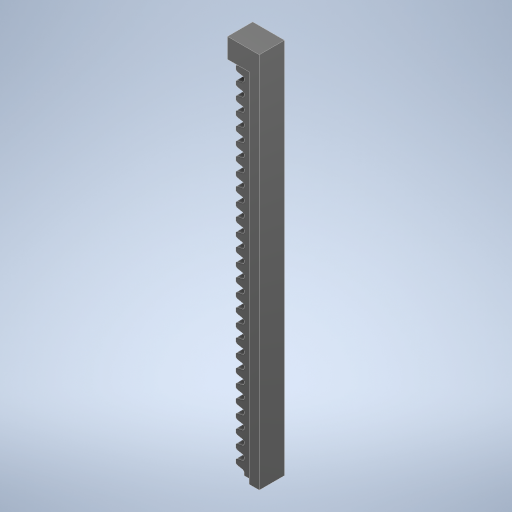
# Autodesk Inventor part: Hreben_Stylus
Saved by Autodesk Inventor 2024.2 (Build 282272000, 272)
## iProperties
Created: 2025-06-02
Part Number: Hreben_Stylus
Material: Termoplastická pryskyřice
Document SubType Name: Modeling
Designer: Elite
Density: 1.28 g/cm^3
Appearance: Hladká – černá
Mass: 4.51235 g
Surface Area: 29.4448 cm^2
Volume: 3.52528 cm^3
Author: Elite
Autodesk Inventor part; units mm, degrees
ref_plane "YZ Plane" through (0, 0, 0) normal (1, 0, 0) x (0, 1, 0)
ref_plane "XZ Plane" through (0, 0, 0) normal (0, 1, 0) x (-1, 0, 0)
ref_plane "XY Plane" through (0, 0, 0) normal (0, 0, 1) x (1, 0, 0)
sketch "Náčrt1" plane through (0, 0, 0) normal (0, 0, 1) x (1, 0, 0)
  line L0 (-2.539999, 6.35) -> (0, 6.35)
  line L1 (-2.539999, 6.35) -> (-3.809999, 5.08)
  line L2 (-3.809999, 5.08) -> (-5.079999, 5.08)
  line L3 (-5.079999, 5.08) -> (-5.079999, 1.27)
  line L4 (-5.079999, 1.27) -> (-3.809999, 1.27)
  line L5 (-3.809999, 1.27) -> (-2.539999, 0)
  line L6 (-2.539999, 0) -> (0, 0)
  line L7 (0, 0) -> (0, 6.35)
  constraints: 16 end point
extrude "Vysunutí1" add sketch "Náčrt1" against normal blind 90
sketch "Náčrt2" plane through (-3.809999, 5.08, 0) normal (0, 1, 0) x (1, 0, 0)
  line L0 (0, 0) -> (-1.27, 0)
  line L1 (0, 0) -> (0, 90)
  line L2 (-1.27, 90) -> (0, 90)
  line L3 (-1.27, 0) -> (-1.27, 90)
  arc A0 (-1.678461, 2.998415) -> (-1.27, 3.497336) centre (-1.778009, 3.496575) ccw
  arc A1 (-2.97646, 2.739034) -> (-3.389, 2.240304) centre (-2.881172, 2.240226) ccw
  arc A2 (-3.389, 1.845748) -> (-2.971901, 1.32351) centre (-2.881505, 1.82339) ccw
  line L4 (-2.990322, 1.327194) -> (-2.971901, 1.32351)
  arc A3 (-1.27, 0.566986) -> (-1.677758, 1.064456) centre (-1.777338, 0.566986) ccw
  line L5 (-1.27, 3.868884) -> (-1.27, 3.495814)
  line L6 (-1.27, 0) -> (-1.27, 90)
  line L7 (-2.971901, 1.32351) -> (-1.677758, 1.064456)
  line L8 (-3.389, 1.845748) -> (-3.389, 2.24059)
  line L9 (-2.97646, 2.739034) -> (-1.678461, 2.998415)
  line L10 (-1.27, 0.566986) -> (-1.27, 3.868884)
  arc A4 (-1.678461, 6.300312) -> (-1.27, 6.799234) centre (-1.778009, 6.798472) ccw
  arc A5 (-2.97646, 6.040931) -> (-3.389, 5.542202) centre (-2.881172, 5.542123) ccw
  arc A6 (-3.389, 5.147645) -> (-2.971901, 4.625407) centre (-2.881505, 5.125287) ccw
  line L11 (-2.990322, 4.629092) -> (-2.971901, 4.625407)
  arc A7 (-1.27, 3.868884) -> (-1.677758, 4.366353) centre (-1.777338, 3.868884) ccw
  line L12 (-1.27, 7.170781) -> (-1.27, 6.797711)
  line L13 (-2.971901, 4.625407) -> (-1.677758, 4.366353)
  line L14 (-3.389, 5.147645) -> (-3.389, 5.542488)
  line L15 (-2.97646, 6.040931) -> (-1.678461, 6.300312)
  line L16 (-1.27, 3.868884) -> (-1.27, 7.170781)
  arc A8 (-1.678461, 9.602209) -> (-1.27, 10.101131) centre (-1.778009, 10.10037) ccw
  arc A9 (-2.97646, 9.342828) -> (-3.389, 8.844099) centre (-2.881172, 8.844021) ccw
  arc A10 (-3.389, 8.449542) -> (-2.971901, 7.927305) centre (-2.881505, 8.427184) ccw
  line L17 (-2.990322, 7.930989) -> (-2.971901, 7.927305)
  arc A11 (-1.27, 7.170781) -> (-1.677758, 7.668251) centre (-1.777338, 7.170781) ccw
  line L18 (-1.27, 10.472678) -> (-1.27, 10.099608)
  line L19 (-2.971901, 7.927305) -> (-1.677758, 7.668251)
  line L20 (-3.389, 8.449542) -> (-3.389, 8.844385)
  line L21 (-2.97646, 9.342828) -> (-1.678461, 9.602209)
  line L22 (-1.27, 7.170781) -> (-1.27, 10.472678)
  arc A12 (-1.678461, 12.904106) -> (-1.27, 13.403028) centre (-1.778009, 13.402267) ccw
  arc A13 (-2.97646, 12.644726) -> (-3.389, 12.145996) centre (-2.881172, 12.145918) ccw
  arc A14 (-3.389, 11.751439) -> (-2.971901, 11.229202) centre (-2.881505, 11.729081) ccw
  line L23 (-2.990322, 11.232886) -> (-2.971901, 11.229202)
  arc A15 (-1.27, 10.472678) -> (-1.677758, 10.970148) centre (-1.777338, 10.472678) ccw
  line L24 (-1.27, 13.774575) -> (-1.27, 13.401505)
  line L25 (-2.971901, 11.229202) -> (-1.677758, 10.970148)
  line L26 (-3.389, 11.751439) -> (-3.389, 12.146282)
  line L27 (-2.97646, 12.644726) -> (-1.678461, 12.904106)
  line L28 (-1.27, 10.472678) -> (-1.27, 13.774575)
  arc A16 (-1.678461, 16.206003) -> (-1.27, 16.704925) centre (-1.778009, 16.704164) ccw
  arc A17 (-2.97646, 15.946623) -> (-3.389, 15.447893) centre (-2.881172, 15.447815) ccw
  arc A18 (-3.389, 15.053337) -> (-2.971901, 14.531099) centre (-2.881505, 15.030979) ccw
  line L29 (-2.990322, 14.534783) -> (-2.971901, 14.531099)
  arc A19 (-1.27, 13.774575) -> (-1.677758, 14.272045) centre (-1.777338, 13.774575) ccw
  line L30 (-1.27, 17.076472) -> (-1.27, 16.703403)
  line L31 (-2.971901, 14.531099) -> (-1.677758, 14.272045)
  line L32 (-3.389, 15.053337) -> (-3.389, 15.448179)
  line L33 (-2.97646, 15.946623) -> (-1.678461, 16.206003)
  line L34 (-1.27, 13.774575) -> (-1.27, 17.076472)
  arc A20 (-1.678461, 19.507901) -> (-1.27, 20.006822) centre (-1.778009, 20.006061) ccw
  arc A21 (-2.97646, 19.24852) -> (-3.389, 18.74979) centre (-2.881172, 18.749712) ccw
  arc A22 (-3.389, 18.355234) -> (-2.971901, 17.832996) centre (-2.881505, 18.332876) ccw
  line L35 (-2.990322, 17.83668) -> (-2.971901, 17.832996)
  arc A23 (-1.27, 17.076472) -> (-1.677758, 17.573942) centre (-1.777338, 17.076472) ccw
  line L36 (-1.27, 20.37837) -> (-1.27, 20.0053)
  line L37 (-2.971901, 17.832996) -> (-1.677758, 17.573942)
  line L38 (-3.389, 18.355234) -> (-3.389, 18.750076)
  line L39 (-2.97646, 19.24852) -> (-1.678461, 19.507901)
  line L40 (-1.27, 17.076472) -> (-1.27, 20.37837)
  arc A24 (-1.678461, 22.809798) -> (-1.27, 23.30872) centre (-1.778009, 23.307958) ccw
  arc A25 (-2.97646, 22.550417) -> (-3.389, 22.051688) centre (-2.881172, 22.051609) ccw
  arc A26 (-3.389, 21.657131) -> (-2.971901, 21.134893) centre (-2.881505, 21.634773) ccw
  line L41 (-2.990322, 21.138578) -> (-2.971901, 21.134893)
  arc A27 (-1.27, 20.37837) -> (-1.677758, 20.875839) centre (-1.777338, 20.37837) ccw
  line L42 (-1.27, 23.680267) -> (-1.27, 23.307197)
  line L43 (-2.971901, 21.134893) -> (-1.677758, 20.875839)
  line L44 (-3.389, 21.657131) -> (-3.389, 22.051974)
  line L45 (-2.97646, 22.550417) -> (-1.678461, 22.809798)
  line L46 (-1.27, 20.37837) -> (-1.27, 23.680267)
  arc A28 (-1.678461, 26.111695) -> (-1.27, 26.610617) centre (-1.778009, 26.609856) ccw
  arc A29 (-2.97646, 25.852314) -> (-3.389, 25.353585) centre (-2.881172, 25.353507) ccw
  arc A30 (-3.389, 24.959028) -> (-2.971901, 24.436791) centre (-2.881505, 24.93667) ccw
  line L47 (-2.990322, 24.440475) -> (-2.971901, 24.436791)
  arc A31 (-1.27, 23.680267) -> (-1.677758, 24.177737) centre (-1.777338, 23.680267) ccw
  line L48 (-1.27, 26.982164) -> (-1.27, 26.609094)
  line L49 (-2.971901, 24.436791) -> (-1.677758, 24.177737)
  line L50 (-3.389, 24.959028) -> (-3.389, 25.353871)
  line L51 (-2.97646, 25.852314) -> (-1.678461, 26.111695)
  line L52 (-1.27, 23.680267) -> (-1.27, 26.982164)
  line L53 (-2.971901, 27.738688) -> (-1.677758, 27.479634)
  line L54 (-2.97646, 29.154212) -> (-1.678461, 29.413592)
  line L55 (-2.990322, 27.742372) -> (-2.971901, 27.738688)
  arc A32 (-2.97646, 29.154212) -> (-3.389, 28.655482) centre (-2.881172, 28.655404) ccw
  line L56 (-3.389, 28.260925) -> (-3.389, 28.655768)
  arc A33 (-3.389, 28.260925) -> (-2.971901, 27.738688) centre (-2.881505, 28.238567) ccw
  arc A34 (-1.27, 26.982164) -> (-1.677758, 27.479634) centre (-1.777338, 26.982164) ccw
  arc A35 (-1.678461, 29.413592) -> (-1.27, 29.912514) centre (-1.778009, 29.911753) ccw
  line L57 (-1.27, 30.284061) -> (-1.27, 29.910991)
  line L58 (-1.27, 26.982164) -> (-1.27, 30.284061)
  line L59 (-2.971901, 31.040585) -> (-1.677758, 30.781531)
  line L60 (-2.97646, 32.456109) -> (-1.678461, 32.715489)
  line L61 (-2.990322, 31.044269) -> (-2.971901, 31.040585)
  arc A36 (-2.97646, 32.456109) -> (-3.389, 31.957379) centre (-2.881172, 31.957301) ccw
  line L62 (-3.389, 31.562823) -> (-3.389, 31.957665)
  arc A37 (-3.389, 31.562823) -> (-2.971901, 31.040585) centre (-2.881505, 31.540465) ccw
  arc A38 (-1.27, 30.284061) -> (-1.677758, 30.781531) centre (-1.777338, 30.284061) ccw
  arc A39 (-1.678461, 32.715489) -> (-1.27, 33.214411) centre (-1.778009, 33.21365) ccw
  line L63 (-1.27, 33.585958) -> (-1.27, 33.212889)
  line L64 (-1.27, 30.284061) -> (-1.27, 33.585958)
  line L65 (-2.971901, 34.342482) -> (-1.677758, 34.083428)
  line L66 (-2.97646, 35.758006) -> (-1.678461, 36.017387)
  line L67 (-2.990322, 34.346166) -> (-2.971901, 34.342482)
  arc A40 (-2.97646, 35.758006) -> (-3.389, 35.259276) centre (-2.881172, 35.259198) ccw
  line L68 (-3.389, 34.86472) -> (-3.389, 35.259562)
  arc A41 (-3.389, 34.86472) -> (-2.971901, 34.342482) centre (-2.881505, 34.842362) ccw
  arc A42 (-1.27, 33.585958) -> (-1.677758, 34.083428) centre (-1.777338, 33.585958) ccw
  arc A43 (-1.678461, 36.017387) -> (-1.27, 36.516308) centre (-1.778009, 36.515547) ccw
  line L69 (-1.27, 36.887856) -> (-1.27, 36.514786)
  line L70 (-1.27, 33.585958) -> (-1.27, 36.887856)
  line L71 (-2.971901, 37.644379) -> (-1.677758, 37.385325)
  line L72 (-2.97646, 39.059903) -> (-1.678461, 39.319284)
  line L73 (-2.990322, 37.648064) -> (-2.971901, 37.644379)
  arc A44 (-2.97646, 39.059903) -> (-3.389, 38.561174) centre (-2.881172, 38.561095) ccw
  line L74 (-3.389, 38.166617) -> (-3.389, 38.56146)
  arc A45 (-3.389, 38.166617) -> (-2.971901, 37.644379) centre (-2.881505, 38.144259) ccw
  arc A46 (-1.27, 36.887856) -> (-1.677758, 37.385325) centre (-1.777338, 36.887856) ccw
  arc A47 (-1.678461, 39.319284) -> (-1.27, 39.818206) centre (-1.778009, 39.817444) ccw
  line L75 (-1.27, 40.189753) -> (-1.27, 39.816683)
  line L76 (-1.27, 36.887856) -> (-1.27, 40.189753)
  line L77 (-2.971901, 40.946276) -> (-1.677758, 40.687223)
  line L78 (-2.97646, 42.3618) -> (-1.678461, 42.621181)
  line L79 (-2.990322, 40.949961) -> (-2.971901, 40.946276)
  arc A48 (-2.97646, 42.3618) -> (-3.389, 41.863071) centre (-2.881172, 41.862993) ccw
  line L80 (-3.389, 41.468514) -> (-3.389, 41.863357)
  arc A49 (-3.389, 41.468514) -> (-2.971901, 40.946276) centre (-2.881505, 41.446156) ccw
  arc A50 (-1.27, 40.189753) -> (-1.677758, 40.687223) centre (-1.777338, 40.189753) ccw
  arc A51 (-1.678461, 42.621181) -> (-1.27, 43.120103) centre (-1.778009, 43.119342) ccw
  line L81 (-1.27, 43.49165) -> (-1.27, 43.11858)
  line L82 (-1.27, 40.189753) -> (-1.27, 43.49165)
  line L83 (-2.971901, 44.248174) -> (-1.677758, 43.98912)
  line L84 (-2.97646, 45.663698) -> (-1.678461, 45.923078)
  line L85 (-2.990322, 44.251858) -> (-2.971901, 44.248174)
  arc A52 (-2.97646, 45.663698) -> (-3.389, 45.164968) centre (-2.881172, 45.16489) ccw
  line L86 (-3.389, 44.770411) -> (-3.389, 45.165254)
  arc A53 (-3.389, 44.770411) -> (-2.971901, 44.248174) centre (-2.881505, 44.748053) ccw
  arc A54 (-1.27, 43.49165) -> (-1.677758, 43.98912) centre (-1.777338, 43.49165) ccw
  arc A55 (-1.678461, 45.923078) -> (-1.27, 46.422) centre (-1.778009, 46.421239) ccw
  line L87 (-1.27, 46.793547) -> (-1.27, 46.420477)
  line L88 (-1.27, 43.49165) -> (-1.27, 46.793547)
  arc A56 (-1.678461, 49.224975) -> (-1.27, 49.723897) centre (-1.778009, 49.723136) ccw
  arc A57 (-2.97646, 48.965595) -> (-3.389, 48.466865) centre (-2.881172, 48.466787) ccw
  arc A58 (-3.389, 48.072309) -> (-2.971901, 47.550071) centre (-2.881505, 48.049951) ccw
  line L89 (-2.990322, 47.553755) -> (-2.971901, 47.550071)
  arc A59 (-1.27, 46.793547) -> (-1.677758, 47.291017) centre (-1.777338, 46.793547) ccw
  line L90 (-1.27, 50.095444) -> (-1.27, 49.722375)
  line L91 (-2.971901, 47.550071) -> (-1.677758, 47.291017)
  line L92 (-3.389, 48.072309) -> (-3.389, 48.467151)
  line L93 (-2.97646, 48.965595) -> (-1.678461, 49.224975)
  line L94 (-1.27, 46.793547) -> (-1.27, 50.095444)
  line L95 (-2.971901, 50.851968) -> (-1.677758, 50.592914)
  line L96 (-2.97646, 52.267492) -> (-1.678461, 52.526873)
  line L97 (-2.990322, 50.855652) -> (-2.971901, 50.851968)
  arc A60 (-2.97646, 52.267492) -> (-3.389, 51.768762) centre (-2.881172, 51.768684) ccw
  line L98 (-3.389, 51.374206) -> (-3.389, 51.769048)
  arc A61 (-3.389, 51.374206) -> (-2.971901, 50.851968) centre (-2.881505, 51.351848) ccw
  arc A62 (-1.27, 50.095444) -> (-1.677758, 50.592914) centre (-1.777338, 50.095444) ccw
  arc A63 (-1.678461, 52.526873) -> (-1.27, 53.025794) centre (-1.778009, 53.025033) ccw
  line L99 (-1.27, 53.397342) -> (-1.27, 53.024272)
  line L100 (-1.27, 50.095444) -> (-1.27, 53.397342)
  line L101 (-2.971901, 54.153865) -> (-1.677758, 53.894811)
  line L102 (-2.97646, 55.569389) -> (-1.678461, 55.82877)
  line L103 (-2.990322, 54.15755) -> (-2.971901, 54.153865)
  arc A64 (-2.97646, 55.569389) -> (-3.389, 55.07066) centre (-2.881172, 55.070581) ccw
  line L104 (-3.389, 54.676103) -> (-3.389, 55.070946)
  arc A65 (-3.389, 54.676103) -> (-2.971901, 54.153865) centre (-2.881505, 54.653745) ccw
  arc A66 (-1.27, 53.397342) -> (-1.677758, 53.894811) centre (-1.777338, 53.397342) ccw
  arc A67 (-1.678461, 55.82877) -> (-1.27, 56.327692) centre (-1.778009, 56.32693) ccw
  line L105 (-1.27, 56.699239) -> (-1.27, 56.326169)
  line L106 (-1.27, 53.397342) -> (-1.27, 56.699239)
  line L107 (-2.971901, 57.455762) -> (-1.677758, 57.196709)
  line L108 (-2.97646, 58.871286) -> (-1.678461, 59.130667)
  line L109 (-2.990322, 57.459447) -> (-2.971901, 57.455762)
  arc A68 (-2.97646, 58.871286) -> (-3.389, 58.372557) centre (-2.881172, 58.372479) ccw
  line L110 (-3.389, 57.978) -> (-3.389, 58.372843)
  arc A69 (-3.389, 57.978) -> (-2.971901, 57.455762) centre (-2.881505, 57.955642) ccw
  arc A70 (-1.27, 56.699239) -> (-1.677758, 57.196709) centre (-1.777338, 56.699239) ccw
  arc A71 (-1.678461, 59.130667) -> (-1.27, 59.629589) centre (-1.778009, 59.628828) ccw
  line L111 (-1.27, 60.001136) -> (-1.27, 59.628066)
  line L112 (-1.27, 56.699239) -> (-1.27, 60.001136)
  line L113 (-2.971901, 60.75766) -> (-1.677758, 60.498606)
  line L114 (-2.97646, 62.173184) -> (-1.678461, 62.432564)
  line L115 (-2.990322, 60.761344) -> (-2.971901, 60.75766)
  arc A72 (-2.97646, 62.173184) -> (-3.389, 61.674454) centre (-2.881172, 61.674376) ccw
  line L116 (-3.389, 61.279897) -> (-3.389, 61.67474)
  arc A73 (-3.389, 61.279897) -> (-2.971901, 60.75766) centre (-2.881505, 61.257539) ccw
  arc A74 (-1.27, 60.001136) -> (-1.677758, 60.498606) centre (-1.777338, 60.001136) ccw
  arc A75 (-1.678461, 62.432564) -> (-1.27, 62.931486) centre (-1.778009, 62.930725) ccw
  line L117 (-1.27, 63.303033) -> (-1.27, 62.929963)
  line L118 (-1.27, 60.001136) -> (-1.27, 63.303033)
  line L119 (-2.971901, 64.059557) -> (-1.677758, 63.800503)
  line L120 (-2.97646, 65.475081) -> (-1.678461, 65.734461)
  line L121 (-2.990322, 64.063241) -> (-2.971901, 64.059557)
  arc A76 (-2.97646, 65.475081) -> (-3.389, 64.976351) centre (-2.881172, 64.976273) ccw
  line L122 (-3.389, 64.581795) -> (-3.389, 64.976637)
  arc A77 (-3.389, 64.581795) -> (-2.971901, 64.059557) centre (-2.881505, 64.559437) ccw
  arc A78 (-1.27, 63.303033) -> (-1.677758, 63.800503) centre (-1.777338, 63.303033) ccw
  arc A79 (-1.678461, 65.734461) -> (-1.27, 66.233383) centre (-1.778009, 66.232622) ccw
  line L123 (-1.27, 66.60493) -> (-1.27, 66.231861)
  line L124 (-1.27, 63.303033) -> (-1.27, 66.60493)
  line L125 (-2.971901, 67.361454) -> (-1.677758, 67.1024)
  line L126 (-2.97646, 68.776978) -> (-1.678461, 69.036358)
  line L127 (-2.990322, 67.365138) -> (-2.971901, 67.361454)
  arc A80 (-2.97646, 68.776978) -> (-3.389, 68.278248) centre (-2.881172, 68.27817) ccw
  line L128 (-3.389, 67.883692) -> (-3.389, 68.278534)
  arc A81 (-3.389, 67.883692) -> (-2.971901, 67.361454) centre (-2.881505, 67.861334) ccw
  arc A82 (-1.27, 66.60493) -> (-1.677758, 67.1024) centre (-1.777338, 66.60493) ccw
  arc A83 (-1.678461, 69.036358) -> (-1.27, 69.53528) centre (-1.778009, 69.534519) ccw
  line L129 (-1.27, 69.906828) -> (-1.27, 69.533758)
  line L130 (-1.27, 66.60493) -> (-1.27, 69.906828)
  arc A84 (-1.678461, 72.338256) -> (-1.27, 72.837178) centre (-1.778009, 72.836416) ccw
  arc A85 (-2.97646, 72.078875) -> (-3.389, 71.580145) centre (-2.881172, 71.580067) ccw
  arc A86 (-3.389, 71.185589) -> (-2.971901, 70.663351) centre (-2.881505, 71.163231) ccw
  line L131 (-2.990322, 70.667035) -> (-2.971901, 70.663351)
  arc A87 (-1.27, 69.906828) -> (-1.677758, 70.404297) centre (-1.777338, 69.906828) ccw
  line L132 (-1.27, 73.208725) -> (-1.27, 72.835655)
  line L133 (-2.971901, 70.663351) -> (-1.677758, 70.404297)
  line L134 (-3.389, 71.185589) -> (-3.389, 71.580432)
  line L135 (-2.97646, 72.078875) -> (-1.678461, 72.338256)
  line L136 (-1.27, 69.906828) -> (-1.27, 73.208725)
  line L137 (-2.971901, 73.965248) -> (-1.677758, 73.706195)
  line L138 (-2.97646, 75.380772) -> (-1.678461, 75.640153)
  line L139 (-2.990322, 73.968933) -> (-2.971901, 73.965248)
  arc A88 (-2.97646, 75.380772) -> (-3.389, 74.882043) centre (-2.881172, 74.881965) ccw
  line L140 (-3.389, 74.487486) -> (-3.389, 74.882329)
  arc A89 (-3.389, 74.487486) -> (-2.971901, 73.965248) centre (-2.881505, 74.465128) ccw
  arc A90 (-1.27, 73.208725) -> (-1.677758, 73.706195) centre (-1.777338, 73.208725) ccw
  arc A91 (-1.678461, 75.640153) -> (-1.27, 76.139075) centre (-1.778009, 76.138314) ccw
  line L141 (-1.27, 76.510622) -> (-1.27, 76.137552)
  line L142 (-1.27, 73.208725) -> (-1.27, 76.510622)
  line L143 (-2.971901, 77.267146) -> (-1.677758, 77.008092)
  line L144 (-2.97646, 78.68267) -> (-1.678461, 78.94205)
  line L145 (-2.990322, 77.27083) -> (-2.971901, 77.267146)
  arc A92 (-2.97646, 78.68267) -> (-3.389, 78.18394) centre (-2.881172, 78.183862) ccw
  line L146 (-3.389, 77.789383) -> (-3.389, 78.184226)
  arc A93 (-3.389, 77.789383) -> (-2.971901, 77.267146) centre (-2.881505, 77.767025) ccw
  arc A94 (-1.27, 76.510622) -> (-1.677758, 77.008092) centre (-1.777338, 76.510622) ccw
  arc A95 (-1.678461, 78.94205) -> (-1.27, 79.440972) centre (-1.778009, 79.440211) ccw
  line L147 (-1.27, 79.812519) -> (-1.27, 79.439449)
  line L148 (-1.27, 76.510622) -> (-1.27, 79.812519)
  line L149 (-2.971901, 80.569043) -> (-1.677758, 80.309989)
  line L150 (-2.97646, 81.984567) -> (-1.678461, 82.243947)
  line L151 (-2.990322, 80.572727) -> (-2.971901, 80.569043)
  arc A96 (-2.97646, 81.984567) -> (-3.389, 81.485837) centre (-2.881172, 81.485759) ccw
  line L152 (-3.389, 81.091281) -> (-3.389, 81.486123)
  arc A97 (-3.389, 81.091281) -> (-2.971901, 80.569043) centre (-2.881505, 81.068923) ccw
  arc A98 (-1.27, 79.812519) -> (-1.677758, 80.309989) centre (-1.777338, 79.812519) ccw
  arc A99 (-1.678461, 82.243947) -> (-1.27, 82.742869) centre (-1.778009, 82.742108) ccw
  line L153 (-1.27, 83.114416) -> (-1.27, 82.741347)
  line L154 (-1.27, 79.812519) -> (-1.27, 83.114416)
  line L155 (-2.971901, 83.87094) -> (-1.677758, 83.611886)
  line L156 (-2.97646, 85.286464) -> (-1.678461, 85.545844)
  line L157 (-2.990322, 83.874624) -> (-2.971901, 83.87094)
  arc A100 (-2.97646, 85.286464) -> (-3.389, 84.787734) centre (-2.881172, 84.787656) ccw
  line L158 (-3.389, 84.393178) -> (-3.389, 84.78802)
  arc A101 (-3.389, 84.393178) -> (-2.971901, 83.87094) centre (-2.881505, 84.37082) ccw
  arc A102 (-1.27, 83.114416) -> (-1.677758, 83.611886) centre (-1.777338, 83.114416) ccw
  arc A103 (-1.678461, 85.545844) -> (-1.27, 86.044766) centre (-1.778009, 86.044005) ccw
  line L159 (-1.27, 86.416314) -> (-1.27, 86.043244)
  line L160 (-1.27, 83.114416) -> (-1.27, 86.416314)
  line L161 (-2.971901, 87.172837) -> (-1.677758, 86.913783)
  line L162 (-2.97646, 88.588361) -> (-1.678461, 88.847742)
  line L163 (-2.990322, 87.176521) -> (-2.971901, 87.172837)
  arc A104 (-2.97646, 88.588361) -> (-3.389, 88.089631) centre (-2.881172, 88.089553) ccw
  line L164 (-3.389, 87.695075) -> (-3.389, 88.089918)
  arc A105 (-3.389, 87.695075) -> (-2.971901, 87.172837) centre (-2.881505, 87.672717) ccw
  arc A106 (-1.27, 86.416314) -> (-1.677758, 86.913783) centre (-1.777338, 86.416314) ccw
  arc A107 (-1.678461, 88.847742) -> (-1.27, 89.346664) centre (-1.778009, 89.345902) ccw
  line L165 (-1.27, 89.718211) -> (-1.27, 89.345141)
  line L166 (-1.27, 86.416314) -> (-1.27, 89.718211)
  point P0 (3.809999, 0)
  point P1 (-1.27, 3.410473)
  point P2 (-3.389, 2.240304)
  point P3 (-1.27, 6.71237)
  point P4 (-1.27, 10.014267)
  point P5 (-1.27, 13.316164)
  point P6 (-1.27, 16.618062)
  point P7 (-1.27, 19.919959)
  point P8 (-1.27, 23.221856)
  point P9 (-1.27, 26.523753)
  point P10 (-1.27, 29.82565)
  point P11 (-1.27, 33.127548)
  point P12 (-1.27, 36.429445)
  point P13 (-1.27, 39.731342)
  point P14 (-1.27, 43.033239)
  point P15 (-1.27, 46.335136)
  point P16 (-1.27, 49.637034)
  point P17 (-1.27, 52.938931)
  point P18 (-1.27, 56.240828)
  point P19 (-1.27, 59.542725)
  point P20 (-1.27, 62.844622)
  point P21 (-1.27, 66.14652)
  point P22 (-1.27, 69.448417)
  point P23 (-1.27, 72.750314)
  point P24 (-1.27, 76.052211)
  point P25 (-1.27, 79.354108)
  point P26 (-1.27, 82.656006)
  point P27 (-1.27, 85.957903)
  point P28 (-1.27, 89.2598)
  point P29 (-3.389, 88.089631)
  point P30 (-3.389, 71.580145)
  point P31 (-3.389, 64.976351)
  point P32 (-3.389, 41.863071)
  point P33 (-1.27, 29.912514)
  point P34 (-3.389, 25.353585)
  point P35 (-3.389, 22.051688)
  point P36 (-3.389, 18.74979)
  point P37 (-3.389, 15.447893)
  point P38 (-3.389, 12.145996)
  point P39 (-3.389, 8.844099)
  point P40 (-3.389, 5.542202)
  constraints: 351 end point, 270 point on circle, 108 centre point, 108 tangent, 29 point on line, 27 collinear, 1 other
sketch "Náčrt2 outline for Vysunutí2" plane through (-3.809999, 5.08, 0) normal (0, 1, 0) x (1, 0, 0)
  line L0 (-2.971901, 1.32351) -> (-1.677758, 1.064456)
  line L1 (-2.990322, 1.327194) -> (-2.971901, 1.32351)
  arc A0 (-3.389, 1.845748) -> (-2.990322, 1.327194) centre (-2.881505, 1.82339) ccw
  line L2 (-3.389, 2.240304) -> (-3.389, 1.845748)
  arc A1 (-2.97646, 2.739034) -> (-3.389, 2.240304) centre (-2.881172, 2.240226) ccw
  line L3 (-1.678461, 2.998415) -> (-2.97646, 2.739034)
  arc A2 (-1.27, 3.497336) -> (-1.678461, 2.998415) centre (-1.778009, 3.496575) cw
  line L4 (-1.27, 0.566986) -> (-1.27, 3.497336)
  arc A3 (-1.677758, 1.064456) -> (-1.27, 0.566986) centre (-1.777338, 0.566986) cw
  line L5 (-2.971901, 87.172837) -> (-1.677758, 86.913783)
  line L6 (-2.990322, 87.176521) -> (-2.971901, 87.172837)
  arc A4 (-3.389, 87.695075) -> (-2.990322, 87.176521) centre (-2.881505, 87.672717) ccw
  line L7 (-3.389, 88.089631) -> (-3.389, 87.695075)
  arc A5 (-2.97646, 88.588361) -> (-3.389, 88.089631) centre (-2.881172, 88.089553) ccw
  line L8 (-1.678461, 88.847742) -> (-2.97646, 88.588361)
  arc A6 (-1.27, 89.346664) -> (-1.678461, 88.847742) centre (-1.778009, 89.345902) cw
  line L9 (-1.27, 86.416314) -> (-1.27, 89.346664)
  arc A7 (-1.677758, 86.913783) -> (-1.27, 86.416314) centre (-1.777338, 86.416314) cw
  line L10 (-2.971901, 83.87094) -> (-1.677758, 83.611886)
  line L11 (-2.990322, 83.874624) -> (-2.971901, 83.87094)
  arc A8 (-3.389, 84.393178) -> (-2.990322, 83.874624) centre (-2.881505, 84.37082) ccw
  line L12 (-3.389, 84.78802) -> (-3.389, 84.393178)
  arc A9 (-2.97646, 85.286464) -> (-3.389, 84.78802) centre (-2.881172, 84.787656) ccw
  line L13 (-1.678461, 85.545844) -> (-2.97646, 85.286464)
  arc A10 (-1.27, 86.044766) -> (-1.678461, 85.545844) centre (-1.778009, 86.044005) cw
  line L14 (-1.27, 83.114416) -> (-1.27, 86.044766)
  arc A11 (-1.677758, 83.611886) -> (-1.27, 83.114416) centre (-1.777338, 83.114416) cw
  line L15 (-2.971901, 80.569043) -> (-1.677758, 80.309989)
  line L16 (-2.990322, 80.572727) -> (-2.971901, 80.569043)
  arc A12 (-3.389, 81.091281) -> (-2.990322, 80.572727) centre (-2.881505, 81.068923) ccw
  line L17 (-3.389, 81.486123) -> (-3.389, 81.091281)
  arc A13 (-2.97646, 81.984567) -> (-3.389, 81.486123) centre (-2.881172, 81.485759) ccw
  line L18 (-1.678461, 82.243947) -> (-2.97646, 81.984567)
  arc A14 (-1.27, 82.742869) -> (-1.678461, 82.243947) centre (-1.778009, 82.742108) cw
  line L19 (-1.27, 79.812519) -> (-1.27, 82.742869)
  arc A15 (-1.677758, 80.309989) -> (-1.27, 79.812519) centre (-1.777338, 79.812519) cw
  line L20 (-2.971901, 77.267146) -> (-1.677758, 77.008092)
  line L21 (-2.990322, 77.27083) -> (-2.971901, 77.267146)
  arc A16 (-3.389, 77.789383) -> (-2.990322, 77.27083) centre (-2.881505, 77.767025) ccw
  line L22 (-3.389, 78.184226) -> (-3.389, 77.789383)
  arc A17 (-2.97646, 78.68267) -> (-3.389, 78.184226) centre (-2.881172, 78.183862) ccw
  line L23 (-1.678461, 78.94205) -> (-2.97646, 78.68267)
  arc A18 (-1.27, 79.440972) -> (-1.678461, 78.94205) centre (-1.778009, 79.440211) cw
  line L24 (-1.27, 76.510622) -> (-1.27, 79.440972)
  arc A19 (-1.677758, 77.008092) -> (-1.27, 76.510622) centre (-1.777338, 76.510622) cw
  line L25 (-2.971901, 73.965248) -> (-1.677758, 73.706195)
  line L26 (-2.990322, 73.968933) -> (-2.971901, 73.965248)
  arc A20 (-3.389, 74.487486) -> (-2.990322, 73.968933) centre (-2.881505, 74.465128) ccw
  line L27 (-3.389, 74.882329) -> (-3.389, 74.487486)
  arc A21 (-2.97646, 75.380772) -> (-3.389, 74.882329) centre (-2.881172, 74.881964) ccw
  line L28 (-1.678461, 75.640153) -> (-2.97646, 75.380772)
  arc A22 (-1.27, 76.139075) -> (-1.678461, 75.640153) centre (-1.778009, 76.138314) cw
  line L29 (-1.27, 73.208725) -> (-1.27, 76.139075)
  arc A23 (-1.677758, 73.706195) -> (-1.27, 73.208725) centre (-1.777338, 73.208725) cw
  line L30 (-2.971901, 70.663351) -> (-1.677758, 70.404297)
  line L31 (-2.990322, 70.667035) -> (-2.971901, 70.663351)
  arc A24 (-3.389, 71.185589) -> (-2.990322, 70.667035) centre (-2.881505, 71.163231) ccw
  line L32 (-3.389, 71.580145) -> (-3.389, 71.185589)
  arc A25 (-2.97646, 72.078875) -> (-3.389, 71.580145) centre (-2.881172, 71.580067) ccw
  line L33 (-1.678461, 72.338256) -> (-2.97646, 72.078875)
  arc A26 (-1.27, 72.837178) -> (-1.678461, 72.338256) centre (-1.778009, 72.836416) cw
  line L34 (-1.27, 69.906828) -> (-1.27, 72.837178)
  arc A27 (-1.677758, 70.404297) -> (-1.27, 69.906828) centre (-1.777338, 69.906828) cw
  line L35 (-2.971901, 67.361454) -> (-1.677758, 67.1024)
  line L36 (-2.990322, 67.365138) -> (-2.971901, 67.361454)
  arc A28 (-3.389, 67.883692) -> (-2.990322, 67.365138) centre (-2.881505, 67.861334) ccw
  line L37 (-3.389, 68.278534) -> (-3.389, 67.883692)
  arc A29 (-2.97646, 68.776978) -> (-3.389, 68.278534) centre (-2.881172, 68.27817) ccw
  line L38 (-1.678461, 69.036358) -> (-2.97646, 68.776978)
  arc A30 (-1.27, 69.53528) -> (-1.678461, 69.036358) centre (-1.778009, 69.534519) cw
  line L39 (-1.27, 66.60493) -> (-1.27, 69.53528)
  arc A31 (-1.677758, 67.1024) -> (-1.27, 66.60493) centre (-1.777338, 66.60493) cw
  line L40 (-2.971901, 64.059557) -> (-1.677758, 63.800503)
  line L41 (-2.990322, 64.063241) -> (-2.971901, 64.059557)
  arc A32 (-3.389, 64.581795) -> (-2.990322, 64.063241) centre (-2.881505, 64.559437) ccw
  line L42 (-3.389, 64.976351) -> (-3.389, 64.581795)
  arc A33 (-2.97646, 65.475081) -> (-3.389, 64.976351) centre (-2.881172, 64.976273) ccw
  line L43 (-1.678461, 65.734461) -> (-2.97646, 65.475081)
  arc A34 (-1.27, 66.233383) -> (-1.678461, 65.734461) centre (-1.778009, 66.232622) cw
  line L44 (-1.27, 63.303033) -> (-1.27, 66.233383)
  arc A35 (-1.677758, 63.800503) -> (-1.27, 63.303033) centre (-1.777338, 63.303033) cw
  line L45 (-2.971901, 60.75766) -> (-1.677758, 60.498606)
  line L46 (-2.990322, 60.761344) -> (-2.971901, 60.75766)
  arc A36 (-3.389, 61.279897) -> (-2.990322, 60.761344) centre (-2.881505, 61.257539) ccw
  line L47 (-3.389, 61.67474) -> (-3.389, 61.279897)
  arc A37 (-2.97646, 62.173184) -> (-3.389, 61.67474) centre (-2.881172, 61.674376) ccw
  line L48 (-1.678461, 62.432564) -> (-2.97646, 62.173184)
  arc A38 (-1.27, 62.931486) -> (-1.678461, 62.432564) centre (-1.778009, 62.930725) cw
  line L49 (-1.27, 60.001136) -> (-1.27, 62.931486)
  arc A39 (-1.677758, 60.498606) -> (-1.27, 60.001136) centre (-1.777338, 60.001136) cw
  line L50 (-2.971901, 57.455762) -> (-1.677758, 57.196709)
  line L51 (-2.990322, 57.459447) -> (-2.971901, 57.455762)
  arc A40 (-3.389, 57.978) -> (-2.990322, 57.459447) centre (-2.881505, 57.955642) ccw
  line L52 (-3.389, 58.372843) -> (-3.389, 57.978)
  arc A41 (-2.97646, 58.871286) -> (-3.389, 58.372843) centre (-2.881172, 58.372478) ccw
  line L53 (-1.678461, 59.130667) -> (-2.97646, 58.871286)
  arc A42 (-1.27, 59.629589) -> (-1.678461, 59.130667) centre (-1.778009, 59.628828) cw
  line L54 (-1.27, 56.699239) -> (-1.27, 59.629589)
  arc A43 (-1.677758, 57.196709) -> (-1.27, 56.699239) centre (-1.777338, 56.699239) cw
  line L55 (-2.971901, 54.153865) -> (-1.677758, 53.894811)
  line L56 (-2.990322, 54.15755) -> (-2.971901, 54.153865)
  arc A44 (-3.389, 54.676103) -> (-2.990322, 54.15755) centre (-2.881505, 54.653745) ccw
  line L57 (-3.389, 55.070946) -> (-3.389, 54.676103)
  arc A45 (-2.97646, 55.569389) -> (-3.389, 55.070946) centre (-2.881172, 55.070581) ccw
  line L58 (-1.678461, 55.82877) -> (-2.97646, 55.569389)
  arc A46 (-1.27, 56.327692) -> (-1.678461, 55.82877) centre (-1.778009, 56.32693) cw
  line L59 (-1.27, 53.397342) -> (-1.27, 56.327692)
  arc A47 (-1.677758, 53.894811) -> (-1.27, 53.397342) centre (-1.777338, 53.397342) cw
  line L60 (-2.971901, 50.851968) -> (-1.677758, 50.592914)
  line L61 (-2.990322, 50.855652) -> (-2.971901, 50.851968)
  arc A48 (-3.389, 51.374206) -> (-2.990322, 50.855652) centre (-2.881505, 51.351848) ccw
  line L62 (-3.389, 51.769048) -> (-3.389, 51.374206)
  arc A49 (-2.97646, 52.267492) -> (-3.389, 51.769048) centre (-2.881172, 51.768684) ccw
  line L63 (-1.678461, 52.526873) -> (-2.97646, 52.267492)
  arc A50 (-1.27, 53.025794) -> (-1.678461, 52.526873) centre (-1.778009, 53.025033) cw
  line L64 (-1.27, 50.095444) -> (-1.27, 53.025794)
  arc A51 (-1.677758, 50.592914) -> (-1.27, 50.095444) centre (-1.777338, 50.095444) cw
  line L65 (-2.971901, 47.550071) -> (-1.677758, 47.291017)
  line L66 (-2.990322, 47.553755) -> (-2.971901, 47.550071)
  arc A52 (-3.389, 48.072309) -> (-2.990322, 47.553755) centre (-2.881505, 48.049951) ccw
  line L67 (-3.389, 48.466865) -> (-3.389, 48.072309)
  arc A53 (-2.97646, 48.965595) -> (-3.389, 48.466865) centre (-2.881172, 48.466787) ccw
  line L68 (-1.678461, 49.224975) -> (-2.97646, 48.965595)
  arc A54 (-1.27, 49.723897) -> (-1.678461, 49.224975) centre (-1.778009, 49.723136) cw
  line L69 (-1.27, 46.793547) -> (-1.27, 49.723897)
  arc A55 (-1.677758, 47.291017) -> (-1.27, 46.793547) centre (-1.777338, 46.793547) cw
  line L70 (-2.971901, 44.248174) -> (-1.677758, 43.98912)
  line L71 (-2.990322, 44.251858) -> (-2.971901, 44.248174)
  arc A56 (-3.389, 44.770411) -> (-2.990322, 44.251858) centre (-2.881505, 44.748053) ccw
  line L72 (-3.389, 45.165254) -> (-3.389, 44.770411)
  arc A57 (-2.97646, 45.663698) -> (-3.389, 45.165254) centre (-2.881172, 45.16489) ccw
  line L73 (-1.678461, 45.923078) -> (-2.97646, 45.663698)
  arc A58 (-1.27, 46.422) -> (-1.678461, 45.923078) centre (-1.778009, 46.421239) cw
  line L74 (-1.27, 43.49165) -> (-1.27, 46.422)
  arc A59 (-1.677758, 43.98912) -> (-1.27, 43.49165) centre (-1.777338, 43.49165) cw
  line L75 (-2.971901, 40.946276) -> (-1.677758, 40.687223)
  line L76 (-2.990322, 40.949961) -> (-2.971901, 40.946276)
  arc A60 (-3.389, 41.468514) -> (-2.990322, 40.949961) centre (-2.881505, 41.446156) ccw
  line L77 (-3.389, 41.863071) -> (-3.389, 41.468514)
  arc A61 (-2.97646, 42.3618) -> (-3.389, 41.863071) centre (-2.881172, 41.862993) ccw
  line L78 (-1.678461, 42.621181) -> (-2.97646, 42.3618)
  arc A62 (-1.27, 43.120103) -> (-1.678461, 42.621181) centre (-1.778009, 43.119342) cw
  line L79 (-1.27, 40.189753) -> (-1.27, 43.120103)
  arc A63 (-1.677758, 40.687223) -> (-1.27, 40.189753) centre (-1.777338, 40.189753) cw
  line L80 (-2.971901, 37.644379) -> (-1.677758, 37.385325)
  line L81 (-2.990322, 37.648064) -> (-2.971901, 37.644379)
  arc A64 (-3.389, 38.166617) -> (-2.990322, 37.648064) centre (-2.881505, 38.144259) ccw
  line L82 (-3.389, 38.56146) -> (-3.389, 38.166617)
  arc A65 (-2.97646, 39.059903) -> (-3.389, 38.56146) centre (-2.881172, 38.561095) ccw
  line L83 (-1.678461, 39.319284) -> (-2.97646, 39.059903)
  arc A66 (-1.27, 39.818206) -> (-1.678461, 39.319284) centre (-1.778009, 39.817444) cw
  line L84 (-1.27, 36.887856) -> (-1.27, 39.818206)
  arc A67 (-1.677758, 37.385325) -> (-1.27, 36.887856) centre (-1.777338, 36.887856) cw
  line L85 (-2.971901, 34.342482) -> (-1.677758, 34.083428)
  line L86 (-2.990322, 34.346166) -> (-2.971901, 34.342482)
  arc A68 (-3.389, 34.86472) -> (-2.990322, 34.346166) centre (-2.881505, 34.842362) ccw
  line L87 (-3.389, 35.259562) -> (-3.389, 34.86472)
  arc A69 (-2.97646, 35.758006) -> (-3.389, 35.259562) centre (-2.881172, 35.259198) ccw
  line L88 (-1.678461, 36.017387) -> (-2.97646, 35.758006)
  arc A70 (-1.27, 36.516308) -> (-1.678461, 36.017387) centre (-1.778009, 36.515547) cw
  line L89 (-1.27, 33.585958) -> (-1.27, 36.516308)
  arc A71 (-1.677758, 34.083428) -> (-1.27, 33.585958) centre (-1.777338, 33.585958) cw
  line L90 (-2.971901, 31.040585) -> (-1.677758, 30.781531)
  line L91 (-2.990322, 31.044269) -> (-2.971901, 31.040585)
  arc A72 (-3.389, 31.562823) -> (-2.990322, 31.044269) centre (-2.881505, 31.540465) ccw
  line L92 (-3.389, 31.957665) -> (-3.389, 31.562823)
  arc A73 (-2.97646, 32.456109) -> (-3.389, 31.957665) centre (-2.881172, 31.957301) ccw
  line L93 (-1.678461, 32.715489) -> (-2.97646, 32.456109)
  arc A74 (-1.27, 33.214411) -> (-1.678461, 32.715489) centre (-1.778009, 33.21365) cw
  line L94 (-1.27, 30.284061) -> (-1.27, 33.214411)
  arc A75 (-1.677758, 30.781531) -> (-1.27, 30.284061) centre (-1.777338, 30.284061) cw
  line L95 (-2.971901, 27.738688) -> (-1.677758, 27.479634)
  line L96 (-2.990322, 27.742372) -> (-2.971901, 27.738688)
  arc A76 (-3.389, 28.260925) -> (-2.990322, 27.742372) centre (-2.881505, 28.238567) ccw
  line L97 (-3.389, 28.655768) -> (-3.389, 28.260925)
  arc A77 (-2.97646, 29.154212) -> (-3.389, 28.655768) centre (-2.881172, 28.655404) ccw
  line L98 (-1.678461, 29.413592) -> (-2.97646, 29.154212)
  arc A78 (-1.27, 29.912514) -> (-1.678461, 29.413592) centre (-1.778009, 29.911753) cw
  line L99 (-1.27, 26.982164) -> (-1.27, 29.912514)
  arc A79 (-1.677758, 27.479634) -> (-1.27, 26.982164) centre (-1.777338, 26.982164) cw
  line L100 (-2.971901, 24.436791) -> (-1.677758, 24.177737)
  line L101 (-2.990322, 24.440475) -> (-2.971901, 24.436791)
  arc A80 (-3.389, 24.959028) -> (-2.990322, 24.440475) centre (-2.881505, 24.93667) ccw
  line L102 (-3.389, 25.353585) -> (-3.389, 24.959028)
  arc A81 (-2.97646, 25.852314) -> (-3.389, 25.353585) centre (-2.881172, 25.353507) ccw
  line L103 (-1.678461, 26.111695) -> (-2.97646, 25.852314)
  arc A82 (-1.27, 26.610617) -> (-1.678461, 26.111695) centre (-1.778009, 26.609856) cw
  line L104 (-1.27, 23.680267) -> (-1.27, 26.610617)
  arc A83 (-1.677758, 24.177737) -> (-1.27, 23.680267) centre (-1.777338, 23.680267) cw
  line L105 (-2.971901, 21.134893) -> (-1.677758, 20.875839)
  line L106 (-2.990322, 21.138578) -> (-2.971901, 21.134893)
  arc A84 (-3.389, 21.657131) -> (-2.990322, 21.138578) centre (-2.881505, 21.634773) ccw
  line L107 (-3.389, 22.051688) -> (-3.389, 21.657131)
  arc A85 (-2.97646, 22.550417) -> (-3.389, 22.051688) centre (-2.881172, 22.051609) ccw
  line L108 (-1.678461, 22.809798) -> (-2.97646, 22.550417)
  arc A86 (-1.27, 23.30872) -> (-1.678461, 22.809798) centre (-1.778009, 23.307958) cw
  line L109 (-1.27, 20.37837) -> (-1.27, 23.30872)
  arc A87 (-1.677758, 20.875839) -> (-1.27, 20.37837) centre (-1.777338, 20.37837) cw
  line L110 (-2.971901, 17.832996) -> (-1.677758, 17.573942)
  line L111 (-2.990322, 17.83668) -> (-2.971901, 17.832996)
  arc A88 (-3.389, 18.355234) -> (-2.990322, 17.83668) centre (-2.881505, 18.332876) ccw
  line L112 (-3.389, 18.74979) -> (-3.389, 18.355234)
  arc A89 (-2.97646, 19.24852) -> (-3.389, 18.74979) centre (-2.881172, 18.749712) ccw
  line L113 (-1.678461, 19.507901) -> (-2.97646, 19.24852)
  arc A90 (-1.27, 20.006822) -> (-1.678461, 19.507901) centre (-1.778009, 20.006061) cw
  line L114 (-1.27, 17.076472) -> (-1.27, 20.006822)
  arc A91 (-1.677758, 17.573942) -> (-1.27, 17.076472) centre (-1.777338, 17.076472) cw
  line L115 (-2.971901, 14.531099) -> (-1.677758, 14.272045)
  line L116 (-2.990322, 14.534783) -> (-2.971901, 14.531099)
  arc A92 (-3.389, 15.053337) -> (-2.990322, 14.534783) centre (-2.881505, 15.030979) ccw
  line L117 (-3.389, 15.447893) -> (-3.389, 15.053337)
  arc A93 (-2.97646, 15.946623) -> (-3.389, 15.447893) centre (-2.881172, 15.447815) ccw
  line L118 (-1.678461, 16.206003) -> (-2.97646, 15.946623)
  arc A94 (-1.27, 16.704925) -> (-1.678461, 16.206003) centre (-1.778009, 16.704164) cw
  line L119 (-1.27, 13.774575) -> (-1.27, 16.704925)
  arc A95 (-1.677758, 14.272045) -> (-1.27, 13.774575) centre (-1.777338, 13.774575) cw
  line L120 (-2.971901, 11.229202) -> (-1.677758, 10.970148)
  line L121 (-2.990322, 11.232886) -> (-2.971901, 11.229202)
  arc A96 (-3.389, 11.751439) -> (-2.990322, 11.232886) centre (-2.881505, 11.729081) ccw
  line L122 (-3.389, 12.145996) -> (-3.389, 11.751439)
  arc A97 (-2.97646, 12.644726) -> (-3.389, 12.145996) centre (-2.881172, 12.145918) ccw
  line L123 (-1.678461, 12.904106) -> (-2.97646, 12.644726)
  arc A98 (-1.27, 13.403028) -> (-1.678461, 12.904106) centre (-1.778009, 13.402267) cw
  line L124 (-1.27, 10.472678) -> (-1.27, 13.403028)
  arc A99 (-1.677758, 10.970148) -> (-1.27, 10.472678) centre (-1.777338, 10.472678) cw
  line L125 (-2.971901, 7.927305) -> (-1.677758, 7.668251)
  line L126 (-2.990322, 7.930989) -> (-2.971901, 7.927305)
  arc A100 (-3.389, 8.449542) -> (-2.990322, 7.930989) centre (-2.881505, 8.427184) ccw
  line L127 (-3.389, 8.844099) -> (-3.389, 8.449542)
  arc A101 (-2.97646, 9.342828) -> (-3.389, 8.844099) centre (-2.881172, 8.844021) ccw
  line L128 (-1.678461, 9.602209) -> (-2.97646, 9.342828)
  arc A102 (-1.27, 10.101131) -> (-1.678461, 9.602209) centre (-1.778009, 10.10037) cw
  line L129 (-1.27, 7.170781) -> (-1.27, 10.101131)
  arc A103 (-1.677758, 7.668251) -> (-1.27, 7.170781) centre (-1.777338, 7.170781) cw
  line L130 (-2.971901, 4.625407) -> (-1.677758, 4.366353)
  line L131 (-2.990322, 4.629092) -> (-2.971901, 4.625407)
  arc A104 (-3.389, 5.147645) -> (-2.990322, 4.629092) centre (-2.881505, 5.125287) ccw
  line L132 (-3.389, 5.542202) -> (-3.389, 5.147645)
  arc A105 (-2.97646, 6.040931) -> (-3.389, 5.542202) centre (-2.881172, 5.542123) ccw
  line L133 (-1.678461, 6.300312) -> (-2.97646, 6.040931)
  arc A106 (-1.27, 6.799234) -> (-1.678461, 6.300312) centre (-1.778009, 6.798472) cw
  line L134 (-1.27, 3.868884) -> (-1.27, 6.799234)
  arc A107 (-1.677758, 4.366353) -> (-1.27, 3.868884) centre (-1.777338, 3.868884) cw
extrude "Vysunutí2" add sketch "Náčrt2 outline for Vysunutí2" against normal up to surface (3.81 mm away)
sketch "Náčrt3" plane through (0, 0, 0) normal (0, 0, 1) x (1, 0, 0)
  line L0 (0, 6.35) -> (-2.539999, 6.35)
  line L1 (0, 6.35) -> (-8, 6.35)
  line L2 (-8, 6.35) -> (-8, 0)
  line L3 (0, 0) -> (-2.539999, 0)
  line L4 (0, 0) -> (0, 6.35)
  line L5 (0, 0) -> (0, 6.35)
  line L6 (0, 0) -> (-8, 0)
  dimension "d4" = 8
  constraints: 8 end point, 1 collinear, 1 horizontal, 1 perpendicular, 1 vertical
  measures "d4" distance of L0.start L1.end
extrude "Vysunutí3" add sketch "Náčrt3" along normal blind 5
chamfer "Zkosení1" [suppressed]
